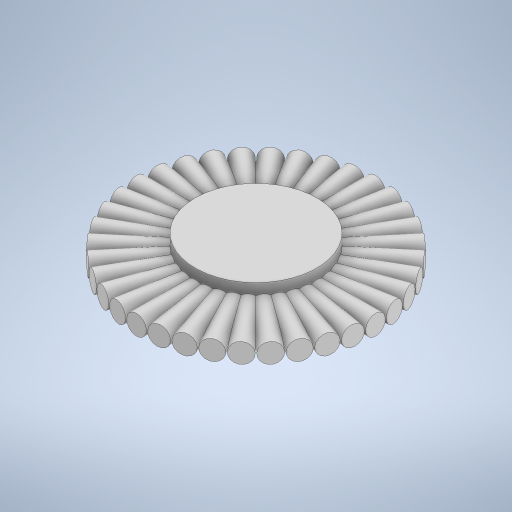
# Autodesk Inventor part: 環形陣列
Saved by Autodesk Inventor 2024.2 (Build 282272000, 272)
## iProperties
Created: 2024-05-02
Part Number: 環形陣列
Material: 一般
Document SubType Name: Modeling
Designer: User
Density: 1 g/cm^3
Appearance: 預設
Author: User
Autodesk Inventor part; units mm, degrees
ref_plane "YZ Plane" through (0, 0, 0) normal (1, 0, 0) x (0, 1, 0)
ref_plane "XZ Plane" through (0, 0, 0) normal (0, 1, 0) x (-1, 0, 0)
ref_plane "XY Plane" through (0, 0, 0) normal (0, 0, 1) x (1, 0, 0)
sketch "草圖1" plane through (0, 0, 0) normal (0, 1, 0) x (-1, 0, 0)
  circle A0 centre (0, 0) radius 15.2723
  constraints: 1 centre point, 1 coincident
extrude "擠出1" add sketch "草圖1" along normal blind 10
sketch "草圖2" plane through (0, 0, 0) normal (1, 0, 0) x (0, 1, 0)
  circle A0 centre (5.0584, 0) radius 2.5
  point P0 (0, 0)
  dimension "d2" = 5
  constraints: 1 centre point
  measures "d2" diameter of A0
extrude "擠出2" add sketch "草圖2" along normal blind 30
pattern_circular "環形陣列1" count 36 over 360 about axis through (0, 0, 0) along (0, 1, 0) of "擠出2"
